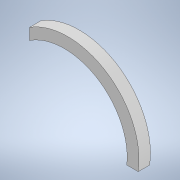
# Autodesk Inventor part: Tube
Saved by Autodesk Inventor 2020 (Build 240168000, 168)
## iProperties
Created: 2021-05-03
Part Number: Tube
Material: Generic
Document SubType Name: Modeling
Designer: chick
Density: 1 g/cm^3
Appearance: Default
Author: chick
Autodesk Inventor part; units mm, degrees
ref_plane "YZ Plane" through (0, 0, 0) normal (1, 0, 0) x (0, 1, 0)
ref_plane "XZ Plane" through (0, 0, 0) normal (0, 1, 0) x (-1, 0, 0)
ref_plane "XY Plane" through (0, 0, 0) normal (0, 0, 1) x (1, 0, 0)
sketch "Sketch1" plane through (0, 0, 0) normal (0, 0, 1) x (1, 0, 0)
  arc A0 (142.8615, 0) -> (0, 92.9819) centre (50.1893, 13.8547) ccw
  arc A1 (127.8615, 0) -> (0, 77.9819) centre (45.5485, 8.851) ccw
  line L0 (0, 92.9819) -> (0, 77.9819)
  line L1 (127.8615, 0) -> (143.5843, 0)
  point P0 (0, 0)
  point P1 (142.8615, 0)
  dimension "d0" = 15
  dimension "d2" = 15
  constraints: 4 end point, 4 point on circle, 2 centre point, 1 vertical
  measures "d0" distance of L0.start L0.end
  measures "d2" distance of A0.start L1.start
extrude "Extrusion1" add sketch "Sketch1" along normal blind 15
body "Solid1"
